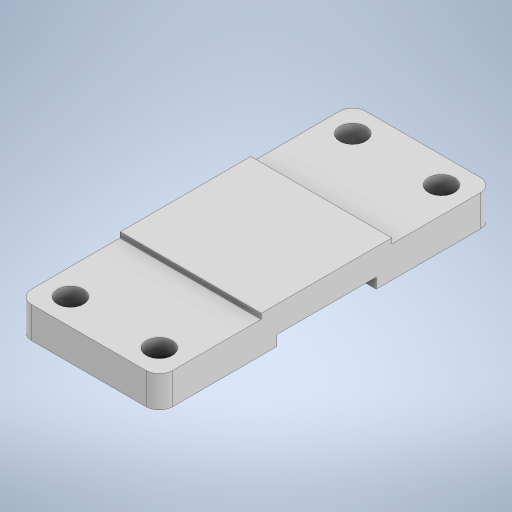
# Autodesk Inventor part: ttab
Saved by Autodesk Inventor 2024 (Build 280153000, 153)
## iProperties
Created: 2024-06-04
Part Number: ttab
Material: Generic
Document SubType Name: Modeling
Designer: Ricsi
Density: 1 g/cm^3
Appearance: Default
Author: Ricsi
Autodesk Inventor part; units mm, degrees
ref_plane "YZ Plane" through (0, 0, 0) normal (1, 0, 0) x (0, 1, 0)
ref_plane "XZ Plane" through (0, 0, 0) normal (0, 1, 0) x (-1, 0, 0)
ref_plane "XY Plane" through (0, 0, 0) normal (0, 0, 1) x (1, 0, 0)
sketch "Sketch1" plane through (0, 0, 0) normal (0, 1, 0) x (-1, 0, 0)
  line L0 (3.6894, 22.9423) -> (-40.3106, 22.9423)
  line L1 (-45.3106, 17.9423) -> (-45.3106, -100.0577)
  line L2 (-40.3106, -105.0577) -> (3.6894, -105.0577)
  line L3 (8.6894, -100.0577) -> (8.6894, 17.9423)
  arc A0 (8.6894, 17.9423) -> (3.6894, 22.9423) centre (3.6894, 17.9423) ccw
  arc A1 (3.6894, -105.0577) -> (8.6894, -100.0577) centre (3.6894, -100.0577) ccw
  arc A2 (-40.3106, 22.9423) -> (-45.3106, 17.9423) centre (-40.3106, 17.9423) ccw
  arc A3 (-45.3106, -100.0577) -> (-40.3106, -105.0577) centre (-40.3106, -100.0577) ccw
  circle A4 centre (-1.3106, 12.9423) radius 5
  circle A5 centre (-1.3106, -95.0577) radius 5
  circle A6 centre (-35.3106, 12.9423) radius 5
  circle A7 centre (-35.3106, -95.0577) radius 5
  point P0 (0, 0)
  point P1 (-45.3106, -105.0577)
  point P2 (-45.3106, 22.9423)
  point P3 (8.6894, -105.0577)
  dimension "d0" = 54
  dimension "d1" = 128
  dimension "d2" = 5
  dimension "d3" = 5
  dimension "d4" = 5
  dimension "d5" = 5
  dimension "d6" = 10
  dimension "d7" = 10
  dimension "d8" = 10
  dimension "d9" = 10
  dimension "d10" = 10
  dimension "d11" = 10
  dimension "d12" = 10
  dimension "d13" = 10
  dimension "d14" = 10
  dimension "d15" = 10
  dimension "d16" = 10
  dimension "d17" = 10
  constraints: 8 centre point, 8 end point, 8 point on circle, 8 tangent, 6 point on line, 2 parallel, 1 horizontal, 1 perpendicular
  measures "d0" distance of point (8.689, -105.058) point (-45.311, -105.058)
  measures "d1" distance of point (-45.311, -105.058) point (-45.311, 22.942)
  measures "d2" radius of A0
  measures "d3" radius of A1
  measures "d4" radius of A2
  measures "d5" radius of A3
  measures "d6" diameter of A4
  measures "d7" diameter of A5
  measures "d8" distance from line of L0 A4.centre
  measures "d9" distance from line of L2 A5.centre
  measures "d10" diameter of A6
  measures "d11" distance from line of L1 A6.centre
  measures "d12" distance from line of L3 A4.centre
  measures "d13" diameter of A7
  measures "d14" distance from line of L2 A7.centre
  measures "d15" distance from line of L1 A7.centre
  measures "d16" distance from line of L3 A5.centre
  measures "d17" distance from line of L0 A6.centre
extrude "Extrusion1" add sketch "Sketch1" along normal blind 12
sketch "Sketch2" plane through (0, 12, 0) normal (0, 1, 0) x (1, 0, 0)
  arc A0 (-8.6894, -17.9423) -> (-3.6894, -22.9423) centre (-3.6894, -17.9423) ccw projected
  line L0 (40.3106, 105.0577) -> (-3.6894, 105.0577) projected
  line L1 (-8.6894, 100.0577) -> (-8.6894, -17.9423) projected
  line L2 (-8.6894, 41.0577) -> (-8.6894, 16.0577)
  line L3 (-8.6894, 41.0577) -> (-8.6894, 66.0577)
  line L4 (-8.6894, 16.0577) -> (45.3106, 16.0577)
  line L5 (45.3106, -17.9423) -> (45.3106, 100.0577) projected
  line L6 (-8.6894, 66.0577) -> (45.3106, 66.0577)
  line L7 (45.3106, 66.0577) -> (45.3106, 16.0577)
  point P0 (0, 0)
  dimension "d21" = 25
  dimension "d22" = 25
  constraints: 10 end point, 3 point on line, 2 horizontal, 1 midpoint, 1 perpendicular
  measures "d21" distance of L2.start L2.end
  measures "d22" distance of L2.start L3.end
extrude "Extrusion2" add sketch "Sketch2" along normal blind 2
sketch "Sketch3" plane through (45.3106, 0, 17.9423) normal (1, 0, 0) x (0, 0, -1)
  line L0 (34, 14) -> (59, 14)
  line L1 (118, 0) -> (0, 0) projected
  line L2 (59, 0) -> (40, 0)
  line L3 (59, 0) -> (78, 0)
  line L4 (40, 0) -> (40, 4)
  line L5 (78, 0) -> (78, 4)
  line L6 (78, 4) -> (40, 4)
  point P0 (17.9423, 0)
  dimension "d26" = 19
  dimension "d27" = 19
  dimension "d28" = 4
  dimension "d29" = 4
  constraints: 12 end point, 2 point on line, 1 midpoint, 1 perpendicular, 1 vertical
  measures "d26" distance of L2.start L2.end
  measures "d27" distance of L2.start L3.end
  measures "d28" distance of L2.end L4.end
  measures "d29" distance of L3.end L5.end
extrude "Extrusion3" cut sketch "Sketch3" against normal blind 54
body "Solid1"
